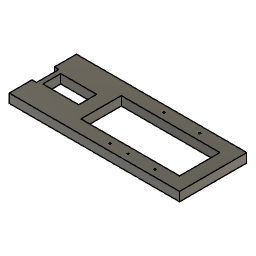
secondbody_prototype1 (Autodesk Fusion 360 design; units mm, degrees)
Autodesk Fusion 360 part; units mm, degrees
sketch "Sketch1" plane through (0, 0, 0) normal (0, 0, 1) x (1, 0, 0)
  line L0 (95, 37.5) -> (-95, 37.5)
  line L1 (-95, 37.5) -> (-95, -37.5)
  line L2 (-95, -37.5) -> (95, -37.5)
  line L3 (95, -37.5) -> (95, 37.5)
  line L4 (95, 37.5) -> (-95, -37.5) construction
  line L5 (-95, 37.5) -> (95, -37.5) construction
  line L6 (-45, 10) -> (-85, 10)
  line L7 (-85, 10) -> (-85, -10)
  line L8 (-85, -10) -> (-45, -10)
  line L9 (-45, -10) -> (-45, 10)
  line L10 (-45, 10) -> (-85, -10) construction
  line L11 (-85, 10) -> (-45, -10) construction
  line L12 (80, 22.5) -> (-30, 22.5)
  line L13 (-30, 22.5) -> (-30, -22.5)
  line L14 (-30, -22.5) -> (80, -22.5)
  line L15 (80, -22.5) -> (80, 22.5)
  line L16 (80, 22.5) -> (-30, -22.5) construction
  line L17 (-30, 22.5) -> (80, -22.5) construction
  line L18 (-90, 13) -> (-106.6701, 13)
  line L19 (-106.6701, 13) -> (-106.6701, -12)
  line L20 (-106.6701, -12) -> (-90, -12)
  line L21 (-90, -12) -> (-90, 13)
  point P0 (-65, 0)
  point P1 (25, 0)
  dimension "d1" = 190
  dimension "d2" = 75
  dimension "d3" = 40
  dimension "d4" = 20
  dimension "d5" = 110
  dimension "d6" = 45
  dimension "d16" = 25
  constraint horizontal L0
  constraint perpendicular L0 L1
  constraint parallel L0 L2
  constraint parallel L1 L3
  constraint coincident L4 origin
  constraint coincident L5 origin
  constraint horizontal L6
  constraint perpendicular L6 L7
  constraint parallel L6 L8
  constraint parallel L7 L9
  constraint coincident L10 P0
  constraint coincident L11 P0
  constraint horizontal L12
  constraint perpendicular L12 L13
  constraint parallel L12 L14
  constraint parallel L13 L15
  constraint coincident L16 P1
  constraint coincident L17 P1
  constraint horizontal L18
  constraint vertical L19
  constraint horizontal L20
  constraint vertical L21
  measures "d1" distance of L1.end L2.end L7
  measures "d2" distance of L0.end L1.end L7
  measures "d3" distance of L7.end L8.end
  measures "d4" distance of L6.end L7.end
  measures "d5" distance of L13.end L14.end
  measures "d6" distance of L12.end L13.end
  measures "d16" distance of L18.start L20.end
extrude "Extrude1" add sketch "Sketch1" along normal blind 10 contours L0 L1 L2 L3 L18 L20 L21 | L1 L18 L20 L21
sketch "Sketch2" plane through (0, 0, 10) normal (0, 0, 1) x (-1, 0, 0)
  line L0 (-80, -22.5) -> (-80, 22.5)
  line L1 (-80, 22.5) -> (30, 22.5)
  line L2 (30, 22.5) -> (30, -22.5)
  line L3 (30, -22.5) -> (-80, -22.5)
  line L4 (45, -10) -> (45, 10)
  line L5 (45, 10) -> (85, 10)
  line L6 (85, 10) -> (85, -10)
  line L7 (85, -10) -> (45, -10)
  line L8 (-95, 37.5) -> (-95, -37.5)
  line L9 (-95, -37.5) -> (95, -37.5)
  line L10 (95, -37.5) -> (95, 37.5)
  line L11 (95, 37.5) -> (-95, 37.5)
  circle A0 centre (-10, -30) radius 1
  circle A1 centre (-50, -30) radius 1
  circle A2 centre (-10, 30) radius 1
  circle A3 centre (-30, 30) radius 1
  circle A4 centre (-60, 30) radius 1
  dimension "d9" = 2
  dimension "d10" = 2
  dimension "d11" = 2
  dimension "d12" = 2
  dimension "d13" = 2
  measures "d9" diameter of A0
  measures "d10" diameter of A1
  measures "d11" diameter of A2
  measures "d12" diameter of A3
  measures "d13" diameter of A4
extrude "Extrude2" cut sketch "Sketch2" against normal blind 30 contours A0 | A1 | A2 | A3 | A4
extrude "Extrude3" cut sketch "Sketch1" along normal blind 40 contours L1 L18 L20 L21 | L1 L18 L19 L20
